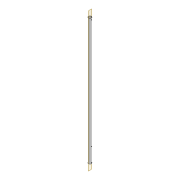
# Autodesk Inventor part: CF_tube_12mm_large
Saved by Autodesk Inventor 2022 (Build 260153000, 153)
## iProperties
Created: 2022-04-28
Part Number: CF_tube_12mm_large
Material: Generic
Document SubType Name: Modeling
Designer: dell
Density: 1 g/cm^3
Appearance: Default
Mass: 10.0217 g
Surface Area: 201.125 cm^2
Volume: 10.0217 cm^3
Author: dell
Autodesk Inventor part; units mm, degrees
ref_plane "XZ Plane" through (0, 0, 0) normal (0, 1, 0) x (-1, 0, 0)
ref_plane "XY Plane" through (0, 0, 0) normal (0, 0, 1) x (1, 0, 0)
sketch "Sketch1" plane through (0, 0, 0) normal (0, 1, 0) x (-1, 0, 0)
  circle A0 centre (0, 0) radius 6
  circle A1 centre (0, 0) radius 5
  dimension "d0" = 12
  dimension "d1" = 10
  constraints: 2 centre point, 2 coincident
  measures "d0" diameter of A0
  measures "d1" diameter of A1
extrude "Extrusion1" add sketch "Sketch1" along normal blind 500
sketch "Sketch2" plane through (0, 0, 0) normal (1, 0, 0) x (0, 1, 0)
  line L0 (0, -6) -> (0, 6) projected
  circle A0 centre (4, 0) radius 1.5
  circle A1 centre (59, 0) radius 1.5
  line L1 (500, -6) -> (500, 6) projected
  circle A2 centre (493.5, 0) radius 1.5
  point P0 (0, 0)
  dimension "d4" = 3
  dimension "d5" = 3
  dimension "d6" = 4
  dimension "d10" = 3
  dimension "d11" = 6.5
  dimension "d12" = 55
  constraints: 3 centre point
  measures "d4" diameter of A0
  measures "d5" diameter of A1
  measures "d6" distance from line of L0 A0.centre
  measures "d10" diameter of A2
  measures "d11" distance from line of L1 A2.centre
  measures "d12" distance of A1.centre A0.centre
extrude "Extrusion2" cut sketch "Sketch2" along normal mid plane 320
body "Solid1"
